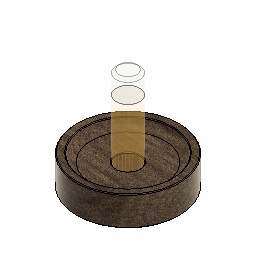
model (Autodesk Fusion 360 design; units mm, degrees)
Autodesk Fusion 360 part; units mm, degrees
sketch "Sketch1" plane through (0, 0, 0) normal (0, 0, 1) x (1, 0, 0)
  circle A0 centre (0, 0) radius 35
  circle A1 centre (0, 0) radius 30
  circle A2 centre (0, 0) radius 8
  dimension "d1" = 16
  dimension "d2" = 60
  dimension "d3" = 70
  constraint coincident A0.centre A1.centre
  constraint concentric A0 A1
  measures "d1" diameter of A2
  measures "d2" diameter of A1
  measures "d3" diameter of A0
extrude "Extrude1" add sketch "Sketch1" along normal blind 20 contours A0 makes body 1
extrude "Extrude2" add sketch "Sketch1" along normal up to surface (14.5 mm away) contours A1 bodies 1
extrude "Extrude3" add sketch "Sketch1" along normal blind 2 contours A2 bodies 1
fillet "Fillet1" radius 5 1 edges at (-27.9698, 10.8485, 14.5) on bodies 1
chamfer "Chamfer1" distance 0.5 angle 45 4 edges at (-27.9698, 10.8485, 20) (-32.6315, -12.6565, 20) (-32.6315, -12.6565, 0) (-7.4586, -2.8929, 14.5) on bodies 1
extrude "Extrude4" add sketch "Sketch1" along normal blind 67 from surface at 2 separate body contours A2 makes body 2
fillet "Fillet2" radius 2 1 edges at (-7.4586, -2.8929, 69) on bodies 2
ref_plane "WorkPlane1" through (0, 0, 54) normal (0, 0, 1) x (1, 0, 0)
split "Split1" by plane through (0, 0, 54) normal (0, 0, 1) bodies 2 makes body 3 at (7.9602, 0.7965, 58.3333)
